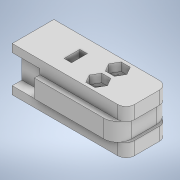
# Autodesk Inventor part: GT2RackB
Saved by Autodesk Inventor 2022 (Build 260153000, 153)
## iProperties
Created: 2022-08-08
Part Number: GT2RackB
Material: Genérico
Document SubType Name: Modeling
Designer: JK
Density: 1 g/cm^3
Appearance: Valor por defecto
Author: JK
Autodesk Inventor part; units mm, degrees
ref_plane "YZ Plane" through (0, 0, 0) normal (1, 0, 0) x (0, 1, 0)
ref_plane "XZ Plane" through (0, 0, 0) normal (0, 1, 0) x (-1, 0, 0)
ref_plane "XY Plane" through (0, 0, 0) normal (0, 0, 1) x (1, 0, 0)
sketch "Boceto1" plane through (0, 0, 0) normal (0, 1, 0) x (-1, 0, 0)
  line L0 (96, 7.5) -> (-96, 7.5)
  line L1 (-96, 7.5) -> (-96, -7.5)
  line L2 (-96, -7.5) -> (96, -7.5)
  line L3 (96, -7.5) -> (96, 7.5)
  line L4 (96, 7.5) -> (-96, -7.5) construction
  line L5 (-96, 7.5) -> (96, -7.5) construction
  point P0 (0, 0)
  dimension "d0" = 192
  dimension "d1" = 15
  constraints: 12 end point, 2 midpoint, 2 parallel, 1 horizontal, 1 perpendicular
  measures "d0" distance between parallel lines of L3 L1
  measures "d1" distance of L2.end L0.start
extrude "Extrusión1" add sketch "Boceto1" along normal blind 10
sketch "Boceto2" plane through (0, 0, 0) normal (1, 0, 0) x (0, 1, 0)
  line L0 (0, 7.5) -> (10, 7.5) projected
  line L1 (1.75, 7.5) -> (8.25, 7.5)
  line L2 (8.25, 7.5) -> (8.25, 9.5)
  line L3 (8.25, 9.5) -> (1.75, 9.5)
  line L4 (1.75, 9.5) -> (1.75, 7.5)
  line L5 (0, -7.5) -> (0, 7.5) projected
  line L6 (0, -7.5) -> (10, -7.5) projected
  line L7 (1.75, -7.5) -> (8.25, -7.5)
  line L8 (8.25, -7.5) -> (8.25, -9.5)
  line L9 (8.25, -9.5) -> (1.75, -9.5)
  line L10 (1.75, -9.5) -> (1.75, -7.5)
  point P0 (0, 0)
  dimension "d4" = 6.5
  dimension "d5" = 1.75
  dimension "d6" = 2
  constraints: 16 end point, 4 parallel, 3 collinear, 2 horizontal, 2 perpendicular, 2 point on line
  measures "d4" distance between parallel lines of L4 L2
  measures "d5" distance between parallel lines of L5 L4
  measures "d6" distance between parallel lines of L0 L3
extrude "Extrusión2" add sketch "Boceto2" along normal mid plane 192
sketch "Boceto4" plane through (-96, 0, -7.5) normal (-1, 0, 0) x (0, 0, 1)
  line L0 (15, 1.75) -> (17, 1.75) projected
  line L1 (0, 8.25) -> (-2, 8.25) projected
  line L2 (17, 1.75) -> (-2, 1.75)
  line L3 (-2, 1.75) -> (-2, 8.25)
  line L4 (-2, 8.25) -> (17, 8.25)
  line L5 (17, 8.25) -> (17, 1.75)
  point P0 (7.5, 0)
  point P1 (15, 1.75)
  point P2 (0, 8.25)
  constraints: 8 end point, 2 parallel, 1 horizontal, 1 perpendicular
extrude "Extrusión3" cut sketch "Boceto4" against normal blind 1
sketch "Boceto5" plane through (96, 0, 7.5) normal (1, 0, 0) x (0, 0, -1)
  line L0 (0, 8.25) -> (-2, 8.25) projected
  line L1 (17, 1.75) -> (17, 8.25) projected
  line L2 (-2, 8.25) -> (17, 8.25)
  line L3 (17, 8.25) -> (17, 1.75)
  line L4 (17, 1.75) -> (-2, 1.75)
  line L5 (-2, 1.75) -> (-2, 8.25)
  point P0 (7.5, 0)
  point P1 (17, 8.25)
  point P2 (0, 8.25)
  constraints: 8 end point, 2 parallel, 1 horizontal, 1 perpendicular
extrude "Extrusión4" cut sketch "Boceto5" against normal blind 1
fillet "Empalme1" radius 5 4 edges at (95, 5, -9.5) (95, 5, 9.5) (-95, 5, -9.5) (-95, 5, 9.5)
fillet "Empalme2" radius 3 8 edges at (96, 9.125, 7.5) (96, 0.875, 7.5) (96, 9.125, -7.5) (96, 0.875, -7.5) (-96, 0.875, 7.5) (-96, 9.125, 7.5) (-96, 0.875, -7.5) (-96, 9.125, -7.5)
sketch "Boceto7" plane through (0, 10, 0) normal (0, 1, 0) x (1, 0, 0)
  line L0 (-90, 9.5) -> (90, 9.5) projected
  line L1 (-90, -9.5) -> (90, -9.5) projected
  line L2 (82.6935, 4) -> (-107.9962, 4)
  line L3 (-107.9962, 4) -> (-107.9962, -4)
  line L4 (-107.9962, -4) -> (82.6935, -4)
  line L5 (82.6935, -4) -> (82.6935, 4)
  line L6 (93, 7.5) -> (-93, 7.5) projected
  line L7 (96, 9.5) -> (75, 9.5)
  line L8 (75, 9.5) -> (75, -22.8831)
  line L9 (75, -22.8831) -> (96, -22.8831)
  line L10 (96, -22.8831) -> (96, 9.5)
  line L11 (96, -4.5) -> (96, 4.5) projected
  line L12 (75, 9.5) -> (65, 9.5)
  line L13 (65, 9.5) -> (65, 4)
  line L14 (65, 4) -> (75, 4)
  line L15 (75, 4) -> (75, 9.5)
  line L16 (75, -9.5) -> (65, -9.5)
  line L17 (65, -9.5) -> (65, -4)
  line L18 (65, -4) -> (75, -4)
  line L19 (75, -4) -> (75, -9.5)
  line L20 (75, 4) -> (55, 4)
  line L21 (55, 4) -> (55, -4)
  line L22 (55, -4) -> (75, -4)
  line L23 (75, -4) -> (75, 4)
  point P0 (75, 4)
  point P1 (75, -4)
  point P2 (55, 4)
  dimension "d17" = 8
  dimension "d18" = 3.5
  dimension "d19" = 21
  dimension "d20" = 10
  dimension "d23" = 10
  constraints: 40 end point, 10 parallel, 5 horizontal, 5 perpendicular, 5 point on line, 4 collinear
  measures "d17" distance of L4.end L2.start
  measures "d18" distance between parallel lines of L6 L2
  measures "d19" distance between parallel lines of L10 L8
  measures "d20" distance between parallel lines of L15 L13
  measures "d23" distance between parallel lines of L13 L21
extrude "Extrusión5" cut sketch "Boceto7" against normal through all contours L0 L8 L6 L13 | L0 L7 L10 L9 L8 L4 L5 L2 | L6 L8 L2 L13 | L2 L8 L4 L21 | L2 L5 L4 L8 | L8 L1 L17 L4 keep common part
sketch "Boceto8" plane through (55, 10, -4) normal (-1, 0, 0) x (0, 0, 1)
  circle A0 centre (4, -5) radius 1.7
  line L0 (0, -10) -> (8, -10) projected
  line L1 (8, 0) -> (8, -10) projected
  point P0 (4, -10)
  dimension "d24" = 3.4
  dimension "d25" = 5
  dimension "d26" = 4
  constraints: 1 centre point
  measures "d24" diameter of A0
  measures "d25" distance from line of A0.centre L0
  measures "d26" distance from line of L1 A0.centre
extrude "Extrusión6" cut sketch "Boceto8" against normal blind 29
sketch "Boceto9" plane through (0, 10, 0) normal (0, 1, 0) x (1, 0, 0)
  line L0 (69, 2.85) -> (71.7, 2.85)
  line L1 (71.7, 2.85) -> (71.7, -2.85)
  line L2 (71.7, -2.85) -> (69, -2.85)
  line L3 (69, -2.85) -> (69, 2.85)
  line L4 (69, 2.85) -> (71.7, -2.85) construction
  line L5 (71.7, 2.85) -> (69, -2.85) construction
  line L6 (65, 4) -> (65, 7.5) projected
  line L7 (96, -4.5) -> (96, 4.5) projected
  point P0 (0, 0)
  point P1 (70.35, 0)
  point P2 (70.35, 0)
  point P3 (96, 0)
  dimension "d29" = 2.7
  dimension "d30" = 5.7
  dimension "d31" = 4
  constraints: 12 end point, 4 midpoint, 2 parallel, 1 horizontal, 1 horizontal alignment, 1 perpendicular
  measures "d29" distance between parallel lines of L1 L3
  measures "d30" distance of L0.end L1.end
  measures "d31" distance between parallel lines of L6 L3
extrude "Extrusión7" cut sketch "Boceto9" against normal blind 15
sketch "Boceto10" plane through (55, 10, -4) normal (-1, 0, 0) x (0, 0, 1)
  line L0 (-3.5, 3) -> (11.5, 3)
  line L1 (11.5, 3) -> (11.5, 0)
  line L2 (11.5, 0) -> (-3.5, 0)
  line L3 (-3.5, 0) -> (-3.5, 3)
  line L4 (-3.5, -10) -> (11.5, -10)
  line L5 (11.5, -10) -> (11.5, -13)
  line L6 (11.5, -13) -> (-3.5, -13)
  line L7 (-3.5, -13) -> (-3.5, -10)
  line L8 (-3.5, 0) -> (-3.5, -1.75) projected
  line L9 (-3.5, -8.25) -> (-3.5, -10) projected
  line L10 (0, -10) -> (8, -10) projected
  line L11 (11.5, -10) -> (11.5, -8.25) projected
  line L12 (11.5, -1.75) -> (11.5, 0) projected
  line L13 (11.5, 0) -> (8, 0) projected
  point P0 (4, -10)
  dimension "d34" = 3
  dimension "d35" = 3
  constraints: 16 end point, 6 collinear, 4 parallel, 2 horizontal, 2 perpendicular
  measures "d34" distance between parallel lines of L0 L2
  measures "d35" distance of L6.end L4.start
extrude "Extrusión8" add sketch "Boceto10" against normal up to surface (41 mm away)
fillet "Empalme3" radius 3 4 edges at (96, -1.5, -7.5) (96, 11.5, -7.5) (96, 11.5, 7.5) (96, -1.5, 7.5)
sketch "Boceto11" plane through (55, 10, 7.5) normal (-1, 0, 0) x (0, 0, 1)
  line L0 (-15, -1.75) -> (-15, 0) projected
  line L1 (-15, 0.15) -> (-11.5, 0.15)
  line L2 (-11.5, 0.15) -> (-11.5, -10.15)
  line L3 (-11.5, -10.15) -> (-15, -10.15)
  line L4 (-15, -10.15) -> (-15, 0.15)
  line L5 (0, -8.25) -> (0, -10) projected
  line L6 (-3.5, 0.15) -> (0, 0.15)
  line L7 (0, 0.15) -> (0, -10.15)
  line L8 (0, -10.15) -> (-3.5, -10.15)
  line L9 (-3.5, -10.15) -> (-3.5, 0.15)
  line L10 (-11.5, 0) -> (-11.5, -10) projected
  line L11 (-3.5, 0) -> (-3.5, -10) projected
  line L12 (-15, 0) -> (-11.5, 0) projected
  line L13 (-11.5, -10) -> (-15, -10) projected
  point P0 (-7.5, -10)
  point P1 (-15, 3)
  point P2 (0, -13)
  point P3 (0, -8.25)
  point P4 (-15, -1.75)
  dimension "d39" = 0.15
  dimension "d40" = 0.15
  constraints: 16 end point, 4 collinear, 4 parallel, 2 horizontal, 2 perpendicular, 2 point on line
  measures "d39" distance between parallel lines of L1 L12
  measures "d40" distance between parallel lines of L13 L3
extrude "Extrusión9" cut sketch "Boceto11" against normal up to surface (10 mm away) contours L0 L12 L2 L13 L4 | L13 L2 L3 L4 | L5 L7 L8 L9 L6
sketch "Boceto12" plane through (55, 13, 7.5) normal (0, 1, 0) x (1, 0, 0)
  circle A0 centre (27, 11) radius 1.7
  circle A1 centre (27, 4) radius 1.7
  line L0 (35, 12) -> (35, 3) projected
  line L1 (0, 15) -> (38, 15) projected
  line L2 (0, 0) -> (0, 15) projected
  line L3 (0, 0) -> (38, 0) projected
  line L4 (41, 3) -> (41, 12) projected
  arc A2 (38, 0) -> (41, 3) centre (38, 3) ccw projected
  arc A3 (41, 12) -> (38, 15) centre (38, 12) ccw projected
  point P0 (-55, 7.5)
  dimension "d43" = 3.4
  dimension "d44" = 3.4
  dimension "d45" = 8
  dimension "d46" = 4
  dimension "d47" = 4
  constraints: 2 centre point, 1 vertical alignment
  measures "d43" diameter of A0
  measures "d44" diameter of A1
  measures "d45" distance from line of L0 A0.centre
  measures "d46" distance from line of L1 A0.centre
  measures "d47" distance from line of L3 A1.centre
extrude "Extrusión10" cut sketch "Boceto12" against normal through all contours A0 | A1
sketch "Boceto13" plane through (55, 13, 7.5) normal (0, 1, 0) x (1, 0, 0)
  line L0 (14, 4.65) -> (14, 10.35) projected
  line L1 (14, 10.35) -> (16.7, 10.35) projected
  line L2 (16.7, 4.65) -> (14, 4.65) projected
  line L3 (16.7, 10.35) -> (16.7, 4.65) projected
  point P0 (-55, 7.5)
extrude "Extrusión11" cut sketch "Boceto13" against normal through all
sketch "Boceto14" plane through (55, 13, 7.5) normal (0, 1, 0) x (1, 0, 0)
  circle A0 centre (27, 4) radius 1.7 projected
  circle A1 centre (27, 4) radius 2.85
  line L0 (23.7091, 4) -> (25.3546, 6.85)
  line L1 (25.3546, 6.85) -> (28.6454, 6.85)
  line L2 (28.6454, 6.85) -> (30.2909, 4)
  line L3 (30.2909, 4) -> (28.6454, 1.15)
  line L4 (28.6454, 1.15) -> (25.3546, 1.15)
  line L5 (25.3546, 1.15) -> (23.7091, 4)
  circle A2 centre (27, 11) radius 1.7 projected
  circle A3 centre (27, 11) radius 2.85
  line L6 (23.7091, 11) -> (25.3546, 13.85)
  line L7 (25.3546, 13.85) -> (28.6454, 13.85)
  line L8 (28.6454, 13.85) -> (30.2909, 11)
  line L9 (30.2909, 11) -> (28.6454, 8.15)
  line L10 (28.6454, 8.15) -> (25.3546, 8.15)
  line L11 (25.3546, 8.15) -> (23.7091, 11)
  line L12 (14, 10.35) -> (16.7, 10.35) projected
  line L13 (16.7, 10.35) -> (16.7, 4.65) projected
  line L14 (16.7, 4.65) -> (14, 4.65) projected
  line L15 (14, 4.65) -> (14, 10.35) projected
  circle A4 centre (27, 4) radius 1.7 projected
  circle A5 centre (27, 11) radius 1.7 projected
  line L16 (0, 15) -> (38, 15) projected
  line L17 (0, 0) -> (0, 15) projected
  line L18 (0, 0) -> (38, 0) projected
  line L19 (41, 3) -> (41, 12) projected
  arc A6 (38, 0) -> (41, 3) centre (38, 3) ccw projected
  arc A7 (41, 12) -> (38, 15) centre (38, 12) ccw projected
  point P0 (-55, 7.5)
  dimension "d52" = 5.7
  constraints: 24 end point, 4 coincident, 2 centre point, 2 parallel, 2 tangent, 1 equal radius, 26 other
  measures "d52" diameter of A1
extrude "Extrusión12" cut sketch "Boceto14" against normal blind 3 contours A0 | A1 | A1 L2 L3 | A1 L1 L2 | L3 L4 A1 | A1 L0 L1 | L4 L5 A1 | A1 L5 L0 | A2 | A3 | A3 L8 L9 | A3 L7 L8 | L9 L10 A3 | A3 L6 L7 | L10 L11 A3 | A3 L11 L6
sketch "Boceto15" plane through (55, 10, -7.5) normal (-1, 0, 0) x (0, 0, 1)
  circle A0 centre (7.5, -5) radius 1.7 projected
  circle A1 centre (7.5, -5) radius 1.3
  point P0 (7.5, -10)
  dimension "d55" = 0.4
  constraints: 1 centre point, 1 coincident
  measures "d55" radial gap between concentric circles of A0 A1
extrude "Extrusión13" add sketch "Boceto15" against normal blind 0.5 contours A1
